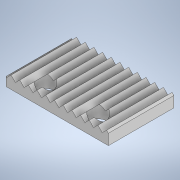
# Autodesk Inventor part: gantryTensioner
Saved by Autodesk Inventor 2020 (Build 240168000, 168)
## iProperties
Created: 2020-02-03
Part Number: gantryTensioner
Material: Generic
Document SubType Name: Modeling
Designer: PAB
Density: 1 g/cm^3
Appearance: Default
Author: PAB
Autodesk Inventor part; units mm, degrees
ref_plane "YZ Plane" through (0, 0, 0) normal (1, 0, 0) x (0, 1, 0)
ref_plane "XZ Plane" through (0, 0, 0) normal (0, 1, 0) x (-1, 0, 0)
ref_plane "XY Plane" through (0, 0, 0) normal (0, 0, 1) x (1, 0, 0)
sketch "Sketch1" plane through (0, 0, 0) normal (0, 1, 0) x (-1, 0, 0)
  line L0 (24, 8) -> (-24, 8)
  line L1 (-24, 8) -> (-24, -8)
  line L2 (-24, -8) -> (24, -8)
  line L3 (24, -8) -> (24, 8)
  point P0 (0, 0)
  dimension "d0" = 48
  dimension "d1" = 16
  constraints: 8 end point, 2 parallel, 1 horizontal, 1 perpendicular
  measures "d0" distance of L2.end L1.end
  measures "d1" distance of L1.end L0.end
extrude "Extrusion1" add sketch "Sketch1" along normal blind 2
sketch "Sketch2" plane through (-24, 0, 8) normal (0, 0, 1) x (1, 0, 0)
  line L0 (0, 2) -> (1.5, 2) construction
  line L1 (0, 3.0607) -> (1.0607, 2)
  line L2 (0, 2) -> (48, 2) projected
  line L3 (0, 3.0607) -> (0, 2)
  line L4 (1.0607, 2) -> (2.1213, 3.0607)
  line L5 (1.0607, 2) -> (2.5607, 2) construction
  line L6 (2.1213, 3.0607) -> (3.182, 2)
  line L7 (3.182, 2) -> (4.2426, 3.0607)
  line L8 (4.2426, 3.0607) -> (5.3033, 2)
  line L9 (5.3033, 2) -> (6.364, 3.0607)
  line L10 (6.364, 3.0607) -> (7.4246, 2)
  line L11 (7.4246, 2) -> (8.4853, 3.0607)
  line L12 (7.4246, 2) -> (8.9246, 2) construction
  line L13 (8.4853, 3.0607) -> (9.5459, 2)
  line L14 (9.5459, 2) -> (10.6066, 3.0607)
  line L15 (10.6066, 3.0607) -> (11.6673, 2)
  line L16 (11.6673, 2) -> (12.7279, 3.0607)
  line L17 (12.7279, 3.0607) -> (13.7886, 2)
  line L18 (13.7886, 2) -> (14.8492, 3.0607)
  line L19 (14.8492, 3.0607) -> (15.9099, 2)
  line L20 (15.9099, 2) -> (16.9706, 3.0607)
  line L21 (16.9706, 3.0607) -> (18.0312, 2)
  line L22 (18.0312, 2) -> (19.0919, 3.0607)
  line L23 (19.0919, 3.0607) -> (20.1525, 2)
  line L24 (20.1525, 2) -> (21.2132, 3.0607)
  line L25 (21.2132, 3.0607) -> (22.2739, 2)
  line L26 (22.2739, 2) -> (23.3345, 3.0607)
  line L27 (23.3345, 3.0607) -> (24.3952, 2)
  line L28 (24.3952, 2) -> (25.4558, 3.0607)
  line L29 (25.4558, 3.0607) -> (26.5165, 2)
  line L30 (26.5165, 2) -> (27.5772, 3.0607)
  line L31 (27.5772, 3.0607) -> (28.6378, 2)
  line L32 (27.5772, 3.0607) -> (29.0772, 3.0607) construction
  line L33 (28.6378, 2) -> (29.6985, 3.0607)
  line L34 (29.6985, 3.0607) -> (30.7591, 2)
  line L35 (30.7591, 2) -> (31.8198, 3.0607)
  line L36 (31.8198, 3.0607) -> (32.8805, 2)
  line L37 (32.8805, 2) -> (33.9411, 3.0607)
  line L38 (33.9411, 3.0607) -> (35.0018, 2)
  line L39 (35.0018, 2) -> (36.0624, 3.0607)
  line L40 (36.0624, 3.0607) -> (37.1231, 2)
  line L41 (37.1231, 2) -> (38.1838, 3.0607)
  line L42 (38.1838, 3.0607) -> (39.2444, 2)
  line L43 (39.2444, 2) -> (40.3051, 3.0607)
  line L44 (40.3051, 3.0607) -> (41.3657, 2)
  line L45 (41.3657, 2) -> (42.4264, 3.0607)
  line L46 (42.4264, 3.0607) -> (43.4871, 2)
  line L47 (43.4871, 2) -> (44.5477, 3.0607)
  line L48 (44.5477, 3.0607) -> (45.6084, 2)
  line L49 (45.6084, 2) -> (46.669, 3.0607)
  line L50 (46.669, 3.0607) -> (47.7297, 2)
  line L51 (47.7297, 2) -> (48.7904, 3.0607)
  line L52 (48, 2) -> (48, 2.2703)
  line L53 (48, 0) -> (48, 2) projected
  line L54 (48, 2) -> (0, 2)
  point P0 (24, 0)
  dimension "d6" = 1.5
  dimension "d7" = 1.5
  dimension "d8" = 45
  dimension "d9" = 1.5
  dimension "d10" = 1.5
  dimension "d11" = 90
  dimension "d12" = 1.5
  dimension "d13" = 1.5
  dimension "d14" = 1.5
  dimension "d15" = 1.5
  dimension "d16" = 45
  dimension "d17" = 1.5
  dimension "d18" = 90
  dimension "d19" = 1.5
  dimension "d20" = 1.5
  dimension "d21" = 1.5
  dimension "d22" = 1.5
  dimension "d23" = 1.5
  dimension "d24" = 1.5
  dimension "d25" = 90
  dimension "d26" = 1.5
  dimension "d27" = 90
  dimension "d28" = 1.5
  dimension "d29" = 90
  dimension "d30" = 1.5
  dimension "d31" = 1.5
  dimension "d32" = 1.5
  dimension "d33" = 1.5
  dimension "d34" = 90
  dimension "d35" = 1.5
  dimension "d36" = 90
  dimension "d37" = 1.5
  dimension "d38" = 90
  dimension "d39" = 1.5
  dimension "d40" = 90
  dimension "d41" = 1.5
  dimension "d42" = 90
  dimension "d43" = 1.5
  dimension "d44" = 90
  dimension "d45" = 1.5
  dimension "d46" = 45
  dimension "d47" = 1.5
  dimension "d48" = 90
  dimension "d49" = 1.5
  dimension "d50" = 90
  dimension "d51" = 1.5
  dimension "d52" = 90
  dimension "d53" = 1.5
  dimension "d54" = 90
  dimension "d55" = 1.5
  dimension "d56" = 90
  dimension "d57" = 1.5
  dimension "d58" = 90
  dimension "d59" = 1.5
  dimension "d60" = 90
  dimension "d61" = 1.5
  dimension "d62" = 90
  dimension "d63" = 1.5
  dimension "d64" = 90
  dimension "d65" = 1.5
  dimension "d66" = 90
  dimension "d67" = 1.5
  dimension "d68" = 90
  dimension "d69" = 1.5
  constraints: 106 end point, 38 perpendicular, 5 horizontal, 3 equal length, 1 point on line, 1 vertical, 8 other
  measures "d6" distance of L1.start L1.end
  measures "d7" distance of L1.end L4.end
  measures "d8" angle of L5 L4
  measures "d9" distance of L4.end L6.end
  measures "d10" distance of L6.end L7.end
  measures "d11" angle of L7 L6
  measures "d12" distance of L7.end L8.end
  measures "d13" distance of L8.end L9.end
  measures "d14" distance of L9.end L10.end
  measures "d15" distance of L10.end L11.end
  measures "d16" angle of L12 L11
  measures "d17" distance of L11.end L13.end
  measures "d18" angle of L11 L13
  measures "d19" distance of L13.end L14.end
  measures "d20" distance of L14.end L15.end
  measures "d21" distance of L15.end L16.end
  measures "d22" distance of L16.end L17.end
  measures "d23" distance of L17.end L18.end
  measures "d24" distance of L18.end L19.end
  measures "d25" angle of L18 L19
  measures "d26" distance of L19.end L20.end
  measures "d27" angle of L20 L19
  measures "d28" distance of L20.end L21.end
  measures "d29" angle of L20 L21
  measures "d30" distance of L21.end L22.end
  measures "d31" distance of L22.end L23.end
  measures "d32" distance of L23.end L24.end
  measures "d33" distance of L24.end L25.end
  measures "d34" angle of L24 L25
  measures "d35" distance of L25.end L26.end
  measures "d36" angle of L26 L25
  measures "d37" distance of L26.end L27.end
  measures "d38" angle of L26 L27
  measures "d39" distance of L27.end L28.end
  measures "d40" angle of L28 L27
  measures "d41" distance of L28.end L29.end
  measures "d42" angle of L28 L29
  measures "d43" distance of L29.end L30.end
  measures "d44" angle of L30 L29
  measures "d45" distance of L30.end L31.end
  measures "d46" angle of L31 L32
  measures "d47" distance of L31.end L33.end
  measures "d48" angle of L33 L31
  measures "d49" distance of L33.end L34.end
  measures "d50" angle of L33 L34
  measures "d51" distance of L34.end L35.end
  measures "d52" angle of L35 L34
  measures "d53" distance of L35.end L36.end
  measures "d54" angle of L35 L36
  measures "d55" distance of L36.end L37.end
  measures "d56" angle of L37 L36
  measures "d57" distance of L37.end L38.end
  measures "d58" angle of L37 L38
  measures "d59" distance of L38.end L39.end
  measures "d60" angle of L39 L38
  measures "d61" distance of L39.end L40.end
  measures "d62" angle of L39 L40
  measures "d63" distance of L40.end L41.end
  measures "d64" angle of L41 L40
  measures "d65" distance of L41.end L42.end
  measures "d66" angle of L41 L42
  measures "d67" distance of L42.end L43.end
  measures "d68" angle of L43 L42
  measures "d69" distance of L43.end L44.end
extrude "Extrusion2" add sketch "Sketch2" against normal blind 16
sketch "Sketch4" plane through (0, 0, 0) normal (0, -1, 0) x (1, 0, 0)
  line L0 (-24, 8) -> (24, 8) projected
  line L1 (12.5, 8) -> (-12.5, 8)
  line L2 (-12.5, 8) -> (-12.5, -8)
  line L3 (-12.5, -8) -> (12.5, -8)
  line L4 (12.5, -8) -> (12.5, 8)
  line L5 (-12.3327, 8) -> (-12.3327, -8) projected
  line L6 (-12.3327, 8) -> (-24, 8)
  line L7 (-24, 8) -> (-24, -8)
  line L8 (-24, -8) -> (-12.3327, -8)
  line L9 (-12.3327, -8) -> (-12.3327, 8)
  line L10 (24, 8) -> (24, -8) projected
  line L11 (12.5, 8) -> (24, 8)
  line L12 (24, 8) -> (24, -8)
  line L13 (24, -8) -> (12.5, -8)
  line L14 (12.5, -8) -> (12.5, 8)
  point P0 (0, 0)
  dimension "d93" = 25
  dimension "d94" = 16
  constraints: 24 end point, 6 parallel, 3 horizontal, 3 perpendicular, 1 point on line
  measures "d93" distance of L3.end L2.end
  measures "d94" distance of L2.end L1.end
extrude "Extrusion4" cut sketch "Sketch4" against normal blind 10 contours L0 L2 L8 L7 | L0 L10 L13 L4
sketch "Sketch5" plane through (0, 0, 0) normal (0, -1, 0) x (1, 0, 0)
  circle A0 centre (6.934, 5) radius 2
  circle A1 centre (-5.934, 5) radius 2
  point P0 (0, 0)
  dimension "d97" = 4
  dimension "d98" = 4
  constraints: 2 centre point
  measures "d97" diameter of A0
  measures "d98" diameter of A1
extrude "Extrusion5" cut sketch "Sketch5" against normal blind 10
body "Solid1"
